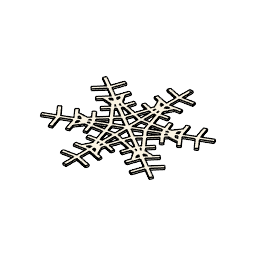
snowflake ornament test (Autodesk Fusion 360 design; units mm, degrees)
part number: 2025-11-13-01-11-33-518
Autodesk Fusion 360 part; units mm, degrees
sketch "Sketch1" plane through (0, 0, 0) normal (0, 1, 0) x (1, 0, 0)
  line L0 (0, 0) -> (0, 12.7)
  line L1 (0, 12.7) -> (0, 25.4)
  line L2 (0, 25.4) -> (0, 38.1)
  line L3 (0, 38.1) -> (0, 50.8)
  line L4 (0, 50.8) -> (0, 63.5)
  line L5 (0, 50.8) -> (-12.7, 53.34)
  line L6 (0, 38.1) -> (-12.7, 40.64)
  line L7 (0, 12.7) -> (-12.7, 15.24)
  line L8 (0, 25.4) -> (-12.7, 27.94)
  line L9 (1.5875, 0) -> (1.5875, 12.7)
  line L10 (1.5875, 12.7) -> (1.5875, 25.4)
  line L11 (1.5875, 25.4) -> (1.5875, 38.1)
  line L12 (1.5875, 38.1) -> (1.5875, 50.8)
  line L13 (1.5875, 50.8) -> (1.5875, 63.5)
  line L14 (-1.5875, 0) -> (-1.5875, 12.7)
  line L15 (-1.5875, 12.7) -> (-1.5875, 25.4)
  line L16 (-1.5875, 25.4) -> (-1.5875, 38.1)
  line L17 (-1.5875, 38.1) -> (-1.5875, 50.8)
  line L18 (-1.5875, 50.8) -> (-1.5875, 63.5)
  line L19 (0.3113, 52.3567) -> (-12.3887, 54.8967)
  line L20 (-0.3113, 49.2433) -> (-13.0113, 51.7833)
  line L21 (-13.0113, 51.7833) -> (-12.7, 53.34)
  line L22 (-12.7, 53.34) -> (-12.3887, 54.8967)
  line L23 (-1.5875, 63.5) -> (1.5875, 63.5)
  line L24 (-1.5875, 0) -> (1.5875, 0)
  line L25 (-12.7, 15.24) -> (-25.4, 17.78)
  line L26 (0.3113, 39.6567) -> (-12.3887, 42.1967)
  line L27 (-0.3113, 36.5433) -> (-13.0113, 39.0833)
  line L28 (0.3113, 26.9567) -> (-12.3887, 29.4967)
  line L29 (-0.3113, 23.8433) -> (-13.0113, 26.3833)
  line L30 (0.3113, 14.2567) -> (-12.3887, 16.7967)
  line L31 (-12.3887, 16.7967) -> (-25.0887, 19.3367)
  line L32 (-0.3113, 11.1433) -> (-13.0113, 13.6833)
  line L33 (-13.0113, 13.6833) -> (-25.7113, 16.2233)
  line L34 (-12.3887, 29.4967) -> (-12.7, 27.94)
  line L35 (-13.0113, 26.3833) -> (-12.7, 27.94)
  line L36 (-12.3887, 42.1967) -> (-12.7, 40.64)
  line L37 (-13.0113, 39.0833) -> (-12.7, 40.64)
  line L38 (-25.4, 17.78) -> (-30.48, 25.4)
  line L39 (-25.4, 17.78) -> (-33.02, 12.7)
  line L40 (-24.0791, 18.6606) -> (-29.1591, 26.2806)
  line L41 (-26.7209, 16.8994) -> (-31.8009, 24.5194)
  line L42 (-26.2806, 19.1009) -> (-33.9006, 14.0209)
  line L43 (-24.5194, 16.4591) -> (-32.1394, 11.3791)
  line L44 (-31.8009, 24.5194) -> (-30.48, 25.4)
  line L45 (-30.48, 25.4) -> (-29.1591, 26.2806)
  line L46 (-33.9006, 14.0209) -> (-33.02, 12.7)
  line L47 (-33.02, 12.7) -> (-32.1394, 11.3791)
  line L48 (-0.3113, 52.3567) -> (12.3887, 54.8967)
  line L49 (0.3113, 49.2433) -> (13.0113, 51.7833)
  line L50 (12.7, 53.34) -> (12.3887, 54.8967)
  line L51 (13.0113, 51.7833) -> (12.7, 53.34)
  line L52 (-0.3113, 39.6567) -> (12.3887, 42.1967)
  line L53 (0.3113, 36.5433) -> (13.0113, 39.0833)
  line L54 (13.0113, 39.0833) -> (12.7, 40.64)
  line L55 (12.3887, 42.1967) -> (12.7, 40.64)
  line L56 (-0.3113, 26.9567) -> (12.3887, 29.4967)
  line L57 (13.0113, 26.3833) -> (12.7, 27.94)
  line L58 (12.3887, 29.4967) -> (12.7, 27.94)
  line L59 (0.3113, 23.8433) -> (13.0113, 26.3833)
  line L60 (12.3887, 16.7967) -> (25.0887, 19.3367)
  line L61 (-0.3113, 14.2567) -> (12.3887, 16.7967)
  line L62 (0.3113, 11.1433) -> (13.0113, 13.6833)
  line L63 (13.0113, 13.6833) -> (25.7113, 16.2233)
  line L64 (24.5194, 16.4591) -> (32.1394, 11.3791)
  line L65 (26.2806, 19.1009) -> (33.9006, 14.0209)
  line L66 (24.0791, 18.6606) -> (29.1591, 26.2806)
  line L67 (26.7209, 16.8994) -> (31.8009, 24.5194)
  line L68 (31.8009, 24.5194) -> (30.48, 25.4)
  line L69 (30.48, 25.4) -> (29.1591, 26.2806)
  line L70 (33.9006, 14.0209) -> (33.02, 12.7)
  line L71 (33.02, 12.7) -> (32.1394, 11.3791)
  line L72 (0, 0) -> (-31.75, 54.9926) construction
  line L73 (0, 0) -> (31.75, 54.9926) construction
  dimension "d1" = 1.5875
  dimension "d2" = -1.5875
  dimension "d3" = 1.5875
  dimension "d4" = -1.5875
  dimension "d5" = 1.5875
  dimension "d6" = -1.5875
  dimension "d7" = 1.5875
  dimension "d8" = -1.5875
  dimension "d9" = 1.5875
  dimension "d10" = -1.5875
  dimension "d12" = 1.5875
  dimension "d13" = -1.5875
  dimension "d14" = 1.5875
  dimension "d15" = -1.5875
  dimension "d20" = 60
  dimension "d21" = 63.5
  dimension "d22" = 63.5
  dimension "d23" = 30
  constraint coincident L0.start L72.start
  constraint vertical L0
  constraint parallel L0 L1
  constraint parallel L1 L2
  constraint parallel L2 L3
  constraint parallel L3 L4
  constraint parallel L5 L6
  constraint parallel L6 L8
  constraint perpendicular L5 L21
  constraint perpendicular L19 L22
  constraint perpendicular L13 L23
  constraint perpendicular L9 L24
  constraint parallel L8 L25
  constraint perpendicular L8 L34
  constraint perpendicular L8 L35
  constraint perpendicular L6 L36
  constraint perpendicular L6 L37
  constraint perpendicular L38 L39
  constraint perpendicular L38 L44
  constraint perpendicular L40 L45
  constraint perpendicular L39 L46
  constraint perpendicular L43 L47
  constraint symmetric L2 L5.end L50.start
  constraint symmetric L2 L6.end L54.end
  constraint symmetric L2 L8.end L57.end
  constraint symmetric L2 L19.start L48.start
  constraint symmetric L2 L19.end L48.end
  constraint symmetric L2 L20.start L49.start
  constraint symmetric L2 L20.end L49.end
  constraint symmetric L2 L26.start L52.start
  constraint symmetric L2 L26.end L52.end
  constraint symmetric L2 L27.start L53.start
  constraint symmetric L2 L27.end L53.end
  constraint symmetric L2 L28.start L56.start
  constraint symmetric L2 L28.end L56.end
  constraint symmetric L2 L29.start L59.start
  constraint symmetric L2 L29.end L57.start
  constraint symmetric L2 L30.start L61.start
  constraint symmetric L2 L30.end L60.start
  constraint symmetric L2 L31.end L60.end
  constraint symmetric L2 L32.start L62.start
  constraint symmetric L2 L32.end L62.end
  constraint symmetric L2 L33.end L63.end
  constraint symmetric L2 L38.end L68.end
  constraint symmetric L2 L39.end L70.end
  constraint symmetric L2 L40.start L66.start
  constraint symmetric L2 L40.end L66.end
  constraint symmetric L2 L41.start L67.start
  constraint symmetric L2 L41.end L67.end
  constraint symmetric L2 L42.start L65.start
  constraint symmetric L2 L42.end L65.end
  constraint symmetric L2 L43.start L64.start
  constraint symmetric L2 L43.end L64.end
  measures "d20" angle of L72 L73
  measures "d21" distance of L0.start L72.end
  measures "d22" distance of L0.start L73.end
  measures "d23" angle of L16 L72
extrude "Extrude2" add sketch "Sketch1" along normal blind 1.5875 makes body 1
pattern_circular "C-Pattern1" count 6 over 360 about axis through (0, 1.75, 0) along (0, 1, 0) of "Extrude2" makes body 2 makes body 3 makes body 4 makes body 5 makes body 6
combine "Combine1" operation add target body 1 tool bodies 6 2 3 5 4
sketch "Sketch2" plane through (0, 0, 0) normal (0, 1, 0) x (1, 0, 0)
  circle A0 centre (0, 61.9125) radius 0.3969
  line L0 (1.5875, 63.5) -> (-1.5875, 63.5)
  line L1 (-1.5875, 63.5) -> (-1.5875, 52.7364)
  dimension "d28" = 0.7937
  dimension "d29" = 1.5875
  dimension "d30" = 1.5875
  measures "d28" diameter of A0
  measures "d29" distance of A0.centre L0
  measures "d30" distance of A0.centre L1
extrude "Extrude3" cut sketch "Sketch2" along normal through all bodies 1
equation "d1 = ( 1 / 16 ) * 1 in"
equation "d2 = -d1"
equation "d3 = ( 1 / 16 ) * 1 in"
equation "d4 = -d3"
equation "d5 = ( 1 / 16 ) * 1 in"
equation "d6 = -d5"
equation "d7 = ( 1 / 16 ) * 1 in"
equation "d8 = -d7"
equation "d9 = ( 1 / 16 ) * 1 in"
equation "d10 = -d9"
equation "d12 = ( 1 / 16 ) * 1 in"
equation "d13 = -d12"
equation "d14 = ( 1 / 16 ) * 1 in"
equation "d15 = -d14"
equation "d24 = ( 1 / 16 ) * 1 in"
equation "d28 = ( 1 / 32 ) * 1 in"
equation "d29 = ( 1 / 16 ) * 1 in"
equation "d30 = ( 1 / 16 ) * 1 in"
